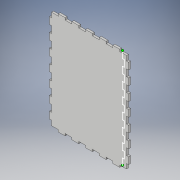
# Autodesk Inventor part: cara_posterior
Saved by Autodesk Inventor 2019 (Build 230136000, 136)
## iProperties
Created: 2018-05-31
Part Number: cara_posterior
Material: Generic
Document SubType Name: Modeling
Designer: seba
Density: 1 g/cm^3
Appearance: Default
Author: seba
Autodesk Inventor part; units mm, degrees
ref_plane "YZ Plane" through (0, 0, 0) normal (1, 0, 0) x (0, 1, 0)
ref_plane "XZ Plane" through (0, 0, 0) normal (0, 1, 0) x (-1, 0, 0)
ref_plane "XY Plane" through (0, 0, 0) normal (0, 0, 1) x (1, 0, 0)
sketch "Sketch1" plane through (0, 0, 0) normal (0, 0, 1) x (1, 0, 0)
  line L0 (311.0517, -16.9965) -> (311.0486, -14.2996) construction
  line L1 (311.0486, -14.2996) -> (302.0591, -14.3097) construction
  line L2 (302.0591, -14.3097) -> (302.0622, -17.0066) construction
  line L3 (302.0622, -17.0066) -> (293.0727, -17.0167) construction
  line L4 (293.0727, -17.0167) -> (293.0696, -14.3199) construction
  line L5 (293.0696, -14.3199) -> (284.0801, -14.33) construction
  line L6 (284.0801, -14.33) -> (284.0832, -17.0268) construction
  line L7 (284.0832, -17.0268) -> (275.0937, -17.0369) construction
  line L8 (275.0937, -17.0369) -> (275.0906, -14.3401) construction
  line L9 (275.0906, -14.3401) -> (266.1012, -14.3502) construction
  line L10 (266.1012, -14.3502) -> (266.1042, -17.047) construction
  line L11 (266.1042, -17.047) -> (257.1147, -17.0571) construction
  line L12 (257.1147, -17.0571) -> (257.1117, -14.3603) construction
  line L13 (257.1117, -14.3603) -> (248.1222, -14.3704) construction
  line L14 (248.1222, -14.3704) -> (248.1252, -17.0672) construction
  line L15 (248.1252, -17.0672) -> (239.1357, -17.0773) construction
  line L16 (239.1357, -17.0773) -> (239.1327, -14.3805) construction
  line L17 (239.1327, -14.3805) -> (230.1432, -14.3906) construction
  line L18 (230.1432, -14.3906) -> (230.1462, -17.0874) construction
  line L19 (320.0411, -23.2891) -> (322.738, -23.2891) construction
  line L20 (322.738, -23.2891) -> (322.738, -32.986) construction
  line L21 (322.738, -32.986) -> (320.0411, -32.986) construction
  line L22 (320.0411, -32.986) -> (320.0411, -41.9755) construction
  line L23 (320.0411, -41.9755) -> (322.738, -41.9755) construction
  line L24 (322.738, -41.9755) -> (322.738, -50.965) construction
  line L25 (322.738, -50.965) -> (320.0411, -50.965) construction
  line L26 (320.0411, -50.965) -> (320.0411, -59.9545) construction
  line L27 (320.0411, -59.9545) -> (322.738, -59.9545) construction
  line L28 (322.738, -59.9545) -> (322.738, -68.944) construction
  line L29 (322.738, -68.944) -> (320.0411, -68.944) construction
  line L30 (320.0411, -68.944) -> (320.0411, -77.9335) construction
  line L31 (320.0411, -77.9335) -> (322.738, -77.9335) construction
  line L32 (322.738, -77.9335) -> (322.738, -86.9229) construction
  line L33 (322.738, -86.9229) -> (320.0411, -86.9229) construction
  line L34 (320.0411, -86.9229) -> (320.0411, -95.9124) construction
  line L35 (320.0411, -95.9124) -> (322.738, -95.9124) construction
  line L36 (322.738, -95.9124) -> (322.738, -104.9019) construction
  line L37 (322.738, -104.9019) -> (320.0411, -104.9019) construction
  line L38 (322.738, -113.8914) -> (323.0503, -123.1532) construction
  line L39 (323.0503, -123.1532) -> (328.4284, -122.9718) construction
  line L40 (328.4284, -122.9718) -> (328.4284, -131.9613) construction
  line L41 (328.4284, -131.9613) -> (331.1252, -131.9613) construction
  line L42 (331.1252, -131.9613) -> (331.1252, -140.9508) construction
  line L43 (331.1252, -140.9508) -> (328.4284, -140.9508) construction
  line L44 (328.4284, -140.9508) -> (328.4284, -147.2435) construction
  line L45 (318.4284, -147.2435) -> (318.4284, -149.9403) construction
  line L46 (318.4284, -149.9403) -> (308.4284, -149.9403) construction
  line L47 (308.4284, -149.9403) -> (308.4284, -147.2435) construction
  line L48 (308.4284, -147.2435) -> (298.4284, -147.2435) construction
  line L49 (298.4284, -147.2435) -> (298.4284, -149.9403) construction
  line L50 (298.4284, -149.9403) -> (288.4284, -149.9403) construction
  line L51 (288.4284, -149.9403) -> (288.4284, -147.2435) construction
  line L52 (288.4284, -147.2435) -> (278.4284, -147.2435) construction
  line L53 (278.4284, -147.2435) -> (278.4284, -149.9403) construction
  line L54 (278.4284, -149.9403) -> (268.4284, -149.9403) construction
  line L55 (268.4284, -149.9403) -> (268.4284, -147.2435) construction
  line L56 (268.4284, -147.2435) -> (258.4284, -147.2435) construction
  line L57 (258.4284, -147.2435) -> (258.4284, -149.9403) construction
  line L58 (258.4284, -149.9403) -> (248.4284, -149.9403) construction
  line L59 (248.4284, -149.9403) -> (248.4284, -147.2435) construction
  line L60 (248.4284, -147.2435) -> (239.4389, -147.2435) construction
  line L61 (239.4389, -147.2435) -> (239.4389, -149.9403) construction
  line L62 (239.4389, -149.9403) -> (230.4494, -149.9403) construction
  line L63 (230.4494, -149.9403) -> (230.4494, -147.2435) construction
  line L64 (218.4599, -140.9508) -> (218.4599, -131.9613) construction
  line L65 (218.4599, -131.9613) -> (221.1567, -131.9613) construction
  line L66 (221.1567, -131.9613) -> (221.1567, -122.9718) construction
  line L67 (221.1567, -122.9718) -> (218.4599, -122.9718) construction
  line L68 (218.4599, -122.9718) -> (218.4599, -113.9823) construction
  line L69 (218.4599, -113.9823) -> (221.1567, -113.9823) construction
  line L70 (221.1567, -113.9823) -> (221.1567, -104.9929) construction
  line L71 (221.1567, -104.9929) -> (218.4599, -104.9929) construction
  line L72 (218.4599, -104.9929) -> (218.4599, -96.0034) construction
  line L73 (218.4599, -96.0034) -> (221.1567, -96.0034) construction
  line L74 (221.1567, -96.0034) -> (221.1567, -87.0139) construction
  line L75 (221.1567, -87.0139) -> (218.4599, -87.0139) construction
  line L76 (218.4599, -87.0139) -> (218.4599, -78.0244) construction
  line L77 (218.4599, -78.0244) -> (221.1567, -78.0244) construction
  line L78 (221.1567, -78.0244) -> (221.1567, -69.0349) construction
  line L79 (221.1567, -69.0349) -> (218.4599, -69.0349) construction
  line L80 (218.4599, -69.0349) -> (218.4599, -60.0454) construction
  line L81 (218.4599, -60.0454) -> (221.1567, -60.0454) construction
  line L82 (221.1567, -60.0454) -> (221.1567, -51.0559) construction
  line L83 (221.1567, -51.0559) -> (218.4599, -51.0559) construction
  line L84 (218.4599, -51.0559) -> (218.4599, -42.0664) construction
  line L85 (218.4599, -42.0664) -> (221.1567, -42.0664) construction
  line L86 (221.1567, -42.0664) -> (221.1567, -33.0769) construction
  line L87 (221.1567, -33.0769) -> (218.4599, -33.0769) construction
  line L88 (218.4599, -33.0769) -> (218.4599, -24.0874) construction
  line L89 (218.4599, -24.0874) -> (221.1567, -24.0874) construction
  line L90 (221.1567, -24.0874) -> (221.1567, -17.0874) construction
  line L91 (320.0411, -104.9019) -> (320.0411, -113.8914) construction
  line L92 (320.0411, -113.8914) -> (322.738, -113.8914) construction
  line L93 (318.4284, -147.2435) -> (328.4284, -147.2435) construction
  line L94 (221.1567, -17.0874) -> (230.1462, -17.0874) construction
  line L95 (221.4599, -147.2435) -> (230.4494, -147.2435) construction
  line L96 (311.0517, -16.9965) -> (320.0411, -16.9965) construction
  line L97 (320.0411, -16.9965) -> (320.0411, -23.2891) construction
  line L98 (221.4599, -147.2435) -> (221.4599, -140.9508) construction
  line L99 (218.4599, -140.9508) -> (221.4599, -140.9508) construction
  line L100 (0, 0) -> (10, 0)
  line L101 (10, 0) -> (10, 3)
  line L102 (10, 3) -> (20, 3)
  line L103 (20, 3) -> (20, 0)
  line L104 (20, 0) -> (30, 0)
  line L105 (30, 0) -> (30, 3)
  line L106 (30, 3) -> (40, 3)
  line L107 (40, 3) -> (40, 0)
  line L108 (40, 0) -> (50, 0)
  line L109 (50, 0) -> (50, 3)
  line L110 (50, 3) -> (60, 3)
  line L111 (60, 3) -> (60, 0)
  line L112 (60, 0) -> (70, 0)
  line L113 (70, 0) -> (70, 3)
  line L114 (70, 3) -> (80, 3)
  line L115 (80, 3) -> (80, 0)
  line L116 (80, 0) -> (90, 0)
  line L117 (90, 0) -> (90, 3)
  line L118 (90, 3) -> (100, 3)
  line L119 (100, 3) -> (100, 0)
  line L120 (100, 0) -> (110, 0)
  line L121 (110, 0) -> (110, -7)
  line L122 (110, -7) -> (113, -7)
  line L123 (113, -7) -> (113, -17)
  line L124 (113, -17) -> (110, -17)
  line L125 (110, -17) -> (110, -27)
  line L126 (110, -27) -> (113, -27)
  line L127 (113, -27) -> (113, -37)
  line L128 (113, -37) -> (110, -37)
  line L129 (110, -37) -> (110, -47)
  line L130 (110, -47) -> (113, -47)
  line L131 (113, -47) -> (113, -57)
  line L132 (113, -57) -> (110, -57)
  line L133 (110, -57) -> (110, -67)
  line L134 (110, -67) -> (113, -67)
  line L135 (113, -67) -> (113, -77)
  line L136 (113, -77) -> (110, -77)
  line L137 (110, -77) -> (110, -87)
  line L138 (110, -87) -> (113, -87)
  line L139 (113, -87) -> (113, -97)
  line L140 (113, -97) -> (110, -97)
  line L141 (110, -97) -> (110, -107)
  line L142 (110, -107) -> (113, -107)
  line L143 (113, -107) -> (113, -117)
  line L144 (113, -117) -> (110, -117)
  line L145 (110, -117) -> (110, -127)
  line L146 (110, -127) -> (113, -127)
  line L147 (113, -127) -> (113, -137)
  line L148 (113, -137) -> (110, -137)
  line L149 (110, -137) -> (110, -144)
  line L150 (110, -144) -> (100, -144)
  line L151 (100, -144) -> (100, -147)
  line L152 (100, -147) -> (90, -147)
  line L153 (90, -147) -> (90, -144)
  line L154 (90, -144) -> (80, -144)
  line L155 (80, -144) -> (80, -147)
  line L156 (80, -147) -> (70, -147)
  line L157 (70, -147) -> (70, -144)
  line L158 (70, -144) -> (60, -144)
  line L159 (60, -144) -> (60, -147)
  line L160 (60, -147) -> (50, -147)
  line L161 (50, -147) -> (50, -144)
  line L162 (50, -144) -> (40, -144)
  line L163 (40, -144) -> (40, -147)
  line L164 (40, -147) -> (30, -147)
  line L165 (30, -147) -> (30, -144)
  line L166 (30, -144) -> (20, -144)
  line L167 (20, -144) -> (20, -147)
  line L168 (20, -147) -> (10, -147)
  line L169 (10, -147) -> (10, -144)
  line L170 (10, -144) -> (0, -144)
  line L171 (0, -144) -> (0, -137)
  line L172 (0, -137) -> (-3, -137)
  line L173 (-3, -137) -> (-3, -127)
  line L174 (-3, -127) -> (0, -127)
  line L175 (0, -127) -> (0, -117)
  line L176 (0, -117) -> (-3, -117)
  line L177 (-3, -117) -> (-3, -107)
  line L178 (-3, -107) -> (0, -107)
  line L179 (0, -107) -> (0, -97)
  line L180 (0, -97) -> (-3, -97)
  line L181 (-3, -97) -> (-3, -87)
  line L182 (-3, -87) -> (0, -87)
  line L183 (0, -87) -> (0, -77)
  line L184 (0, -77) -> (-3, -77)
  line L185 (-3, -77) -> (-3, -67)
  line L186 (-3, -67) -> (0, -67)
  line L187 (0, -67) -> (0, -57)
  line L188 (0, -57) -> (-3, -57)
  line L189 (-3, -57) -> (-3, -47)
  line L190 (-3, -47) -> (0, -47)
  line L191 (0, -47) -> (0, -37)
  line L192 (0, -37) -> (-3, -37)
  line L193 (-3, -37) -> (-3, -27)
  line L194 (-3, -27) -> (0, -27)
  line L195 (0, -27) -> (0, -17)
  line L196 (0, -17) -> (-3, -17)
  line L197 (-3, -17) -> (-3, -7)
  line L198 (-3, -7) -> (0, -7)
  line L199 (0, -7) -> (0, 0)
  dimension "d263" = 8.9895
  dimension "d264" = 7
  dimension "d265" = 10
  dimension "d266" = 3
  dimension "d267" = 10
  dimension "d268" = 10
  dimension "d269" = 10
  dimension "d270" = 10
  dimension "d271" = 10
  dimension "d272" = 10
  dimension "d273" = 10
  dimension "d274" = 10
  dimension "d275" = 10
  dimension "d276" = 10
  dimension "d277" = 7
  dimension "d278" = 3
  dimension "d279" = 10
  dimension "d280" = 10
  dimension "d281" = 10
  dimension "d282" = 10
  dimension "d283" = 10
  dimension "d284" = 10
  dimension "d285" = 10
  dimension "d286" = 10
  dimension "d287" = 10
  dimension "d288" = 10
  dimension "d289" = 10
  dimension "d290" = 10
  dimension "d291" = 10
  dimension "d292" = 7
  dimension "d293" = 3
  dimension "d294" = 3
  dimension "d295" = 110
  dimension "d296" = 144
  dimension "d297" = 3
  dimension "d298" = 3
  dimension "d299" = 3
  dimension "d300" = 3
  dimension "d301" = 3
  constraints: 400 end point, 132 point on line, 108 perpendicular, 14 horizontal, 14 vertical
  measures "d263" distance of L90.end L18.end
  measures "d264" distance of L89.end L90.end
  measures "d265" distance of L100.start L100.end
  measures "d266" distance of L100.end L101.end
  measures "d267" distance of L101.end L102.end
  measures "d268" distance of L103.end L104.end
  measures "d269" distance of L105.end L106.end
  measures "d270" distance of L107.end L108.end
  measures "d271" distance of L109.end L110.end
  measures "d272" distance of L111.end L112.end
  measures "d273" distance of L113.end L114.end
  measures "d274" distance of L115.end L116.end
  measures "d275" distance of L117.end L118.end
  measures "d276" distance of L119.end L120.end
  measures "d277" distance of L120.end L121.end
  measures "d278" distance of L121.end L122.end
  measures "d279" distance of L122.end L123.end
  measures "d280" distance of L124.end L125.end
  measures "d281" distance of L126.end L127.end
  measures "d282" distance of L128.end L129.end
  measures "d283" distance of L130.end L131.end
  measures "d284" distance of L132.end L133.end
  measures "d285" distance of L134.end L135.end
  measures "d286" distance of L136.end L137.end
  measures "d287" distance of L138.end L139.end
  measures "d288" distance of L140.end L141.end
  measures "d289" distance of L142.end L143.end
  measures "d290" distance of L144.end L145.end
  measures "d291" distance of L146.end L147.end
  measures "d292" distance of L148.end L149.end
  measures "d293" distance of L150.end L151.end
  measures "d294" distance of L171.end L172.end
  measures "d295" distance of L120.end L100.start
  measures "d296" distance of L170.end L100.start
  measures "d297" distance of L197.end L198.end
  measures "d298" distance of L179.end L180.end
  measures "d299" distance of L158.end L159.end
  measures "d300" distance of L166.end L167.end
  measures "d301" distance of L110.end L111.end
extrude "Extrusion1" add sketch "Sketch1" along normal blind 3
body "Solid1"
